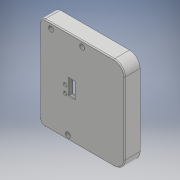
# Autodesk Inventor part: back
Saved by Autodesk Inventor 2017 (Build 210142000, 142)
## iProperties
Created: 2017-07-30
Part Number: back
Material: Generic
Document SubType Name: Modeling
Designer: Käyttäjä
Density: 1 g/cm^3
Appearance: Default
Author: Käyttäjä
Autodesk Inventor part; units mm, degrees
ref_plane "YZ Plane" through (0, 0, 0) normal (1, 0, 0) x (0, 1, 0)
ref_plane "XZ Plane" through (0, 0, 0) normal (0, 1, 0) x (-1, 0, 0)
ref_plane "XY Plane" through (0, 0, 0) normal (0, 0, 1) x (1, 0, 0)
sketch "Sketch1" plane through (0, 0, 0) normal (0, 1, 0) x (-1, 0, 0)
  line L0 (10, 0) -> (83, 0)
  line L1 (87, -4) -> (87, -92)
  line L2 (83, -96) -> (10, -96)
  line L3 (0, -86) -> (0, -10)
  arc A0 (10, 0) -> (0, -10) centre (10, -10) ccw
  arc A1 (0, -86) -> (10, -96) centre (10, -86) ccw
  arc A2 (87, -4) -> (83, 0) centre (83, -4) ccw
  arc A3 (83, -96) -> (87, -92) centre (83, -92) ccw
  line L4 (88.2, -92) -> (88.2, -4)
  arc A4 (88.2, -4) -> (83, 1.2) centre (83, -4) ccw
  line L5 (83, 1.2) -> (10, 1.2)
  arc A5 (10, 1.2) -> (-1.2, -10) centre (10, -10) ccw
  line L6 (-1.2, -10) -> (-1.2, -86)
  arc A6 (-1.2, -86) -> (10, -97.2) centre (10, -86) ccw
  line L7 (10, -97.2) -> (83, -97.2)
  arc A7 (83, -97.2) -> (88.2, -92) centre (83, -92) ccw
  point P0 (0, 0)
  point P1 (87, 0)
  point P2 (0, -96)
  dimension "d0" = 96
  dimension "d1" = 87
  dimension "d2" = 10
  dimension "d3" = 4
  dimension "d4" = 1.2
  constraints: 16 end point, 16 point on circle, 8 centre point, 8 tangent, 6 point on line, 4 parallel, 2 equal radius, 2 perpendicular, 1 horizontal, 7 other
  measures "d0" distance of point (0, -96) point (0, 0)
  measures "d1" distance of point (0, 0) point (87, 0)
  measures "d2" radius of A0
  measures "d3" radius of A2
  measures "d4" distance between parallel lines of L1 L4
extrude "walls" add sketch "Sketch1" along normal blind 15.5
sketch "Sketch2" plane through (0, 0, 0) normal (0, -1, 0) x (1, 0, 0)
  arc A0 (-83, 0) -> (-87, -4) centre (-83, -4) ccw projected
  line L0 (-83, 0) -> (-10, 0) projected
  arc A1 (0, -10) -> (-10, 0) centre (-10, -10) ccw projected
  line L1 (0, -10) -> (0, -86) projected
  arc A2 (-10, -96) -> (0, -86) centre (-10, -86) ccw projected
  line L2 (-10, -96) -> (-83, -96) projected
  arc A3 (-87, -92) -> (-83, -96) centre (-83, -92) ccw projected
  line L3 (-87, -92) -> (-87, -4) projected
  line L4 (-88.2, -92) -> (-88.2, -4) projected
  arc A4 (-88.2, -92) -> (-83, -97.2) centre (-83, -92) ccw projected
  line L5 (-10, -97.2) -> (-83, -97.2) projected
  arc A5 (-10, -97.2) -> (1.2, -86) centre (-10, -86) ccw projected
  line L6 (1.2, -10) -> (1.2, -86) projected
  arc A6 (1.2, -10) -> (-10, 1.2) centre (-10, -10) ccw projected
  line L7 (-83, 1.2) -> (-10, 1.2) projected
  arc A7 (-83, 1.2) -> (-88.2, -4) centre (-83, -4) ccw projected
  point P0 (0, 0)
extrude "back" add sketch "Sketch2" along normal blind 1 contours L0 A1 L1 A2 L2 A3 L3 A0 | L4 A7 L7 A6 L6 A5 L5 A4
sketch "Sketch3" plane through (-88.2, 15.5, -92) normal (-1, 0, 0) x (0, 0, 1)
  line L0 (0, -15.5) -> (88, -15.5) projected
  line L1 (92, -15.5) -> (92, 0) projected
  circle A0 centre (88, -5) radius 2
  line L2 (-4, -15.5) -> (-4, 0) projected
  circle A1 centre (0, -5) radius 2
  dimension "d9" = 4
  dimension "d10" = 4
  dimension "d11" = 10.5
  dimension "d12" = 4
  constraints: 2 centre point, 1 equal radius, 1 horizontal alignment
  measures "d9" distance from line of L1 A0.centre
  measures "d10" distance from line of A1.centre L2
  measures "d11" distance from line of L0 A0.centre
  measures "d12" diameter of A0
extrude "string holes" cut sketch "Sketch3" against normal up to next
sketch "Sketch5" plane through (0, 0, 0) normal (0, 1, 0) x (1, 0, 0)
  circle A0 centre (-76.5, 4.5) radius 2.75
  circle A1 centre (-58.5, 92.5) radius 2.75
  line L0 (0, 86) -> (0, 10) projected
  line L1 (-83, 96) -> (-10, 96) projected
  circle A2 centre (-43.5, 4.5) radius 2.75
  line L2 (-87, 4) -> (-87, 92) projected
  point P0 (0, 0)
  dimension "d19" = 5.5
  dimension "d22" = 3.5
  dimension "d23" = 91.5
  dimension "d130" = 10.5
  dimension "d131" = 33
  dimension "d132" = 15
  constraints: 3 centre point, 2 equal radius, 1 horizontal alignment
  measures "d19" diameter of A0
  measures "d22" distance from line of L1 A1.centre
  measures "d23" distance from line of A0.centre L1
  measures "d130" distance from line of L2 A0.centre
  measures "d131" distance of A2.centre A0.centre
  measures "d132" horizontal distance of A2.centre A1.centre
extrude "PCB pillars" add sketch "Sketch5" along normal blind 10.5
sketch "Sketch6" plane through (-10, 15.5, -97.2) normal (0, 0, -1) x (-1, 0, 0)
  line L0 (45, 0) -> (30, 0)
  line L1 (30, 0) -> (30, -8.5)
  line L2 (30, -8.5) -> (45, -8.5)
  line L3 (45, -8.5) -> (45, 0)
  line L4 (-10, -15.5) -> (-10, 0) projected
  line L5 (0, 0) -> (73, 0) projected
  line L6 (0, -15.5) -> (73, -15.5) projected
  line L7 (77, -15.5) -> (77, -7) projected
  dimension "d30" = 7
  dimension "d137" = 15
  dimension "d138" = 32
  constraints: 8 end point, 2 parallel, 1 horizontal, 1 perpendicular, 1 point on line
  measures "d30" distance between parallel lines of L2 L6
  measures "d137" distance of L1.end L2.end
  measures "d138" distance between parallel lines of L7 L3
sketch "Sketch7" plane through (-76.5, 10.5, -4.5) normal (0, 1, 0) x (1, 0, 0)
  circle A0 centre (0, 0) radius 2.75 projected
  circle A1 centre (0, 0) radius 1.75
  circle A2 centre (33, 0) radius 2.75 projected
  circle A3 centre (18, 88) radius 2.75 projected
  circle A4 centre (33, 0) radius 1.75
  circle A5 centre (18, 88) radius 1.75
  point P0 (76.5, -4.5)
  dimension "d31" = 3.5
  constraints: 3 centre point, 3 coincident, 2 equal radius
  measures "d31" diameter of A1
sketch "Sketch8" plane through (-88.2, 15.5, -92) normal (-1, 0, 0) x (0, 0, 1)
  line L0 (-4, -15.5) -> (-4, 0) projected
  line L1 (92, -15.5) -> (92, 0) projected
  line L2 (88, 0) -> (0, 0) projected
  line L3 (39, 0) -> (49, 0)
  line L4 (49, 0) -> (49, -10.1)
  line L5 (49, -10.1) -> (39, -10.1)
  line L6 (39, -10.1) -> (39, 0)
  line L7 (0, -15.5) -> (88, -15.5) projected
  point P0 (44, -15.5)
  point P1 (44, -10.1)
  dimension "d34" = 5.4
  dimension "d35" = 10
  constraints: 8 end point, 2 midpoint, 2 parallel, 1 horizontal, 1 perpendicular, 1 point on line, 1 vertical alignment
  measures "d34" distance between parallel lines of L7 L5
  measures "d35" distance of L4.end L5.end
extrude "Extrusion5" cut sketch "Sketch8" against normal blind 9.5
extrude "Extrusion6" cut sketch "Sketch7" against normal through all contours A1 | A4 | A5
sketch "Sketch9" plane through (0, 0, 0) normal (0, 1, 0) x (1, 0, 0)
  circle A0 centre (-76.5, 4.5) radius 1.75 projected
  circle A1 centre (-43.5, 4.5) radius 1.75 projected
  circle A2 centre (-58.5, 92.5) radius 1.75 projected
  circle A3 centre (-58.5, 92.5) radius 2.75 projected
  circle A4 centre (-76.5, 4.5) radius 2.75 projected
  circle A5 centre (-43.5, 4.5) radius 2.75 projected
  arc A6 (-87, 4) -> (-83, 0) centre (-83, 4) ccw projected
  line L0 (-83, 0) -> (-10, 0) projected
  arc A7 (-10, 0) -> (0, 10) centre (-10, 10) ccw projected
  line L1 (0, 10) -> (0, 86) projected
  arc A8 (0, 86) -> (-10, 96) centre (-10, 86) ccw projected
  line L2 (-10, 96) -> (-83, 96) projected
  arc A9 (-83, 96) -> (-87, 92) centre (-83, 92) ccw projected
  line L3 (-87, 92) -> (-87, 4) projected
  circle A10 centre (-43.5, 4.5) radius 2.75 projected
  circle A11 centre (-58.5, 92.5) radius 2.75 projected
  circle A12 centre (-76.5, 4.5) radius 5.7
  line L4 (-10, 0) -> (-83, 0) projected
  circle A13 centre (-43.5, 4.5) radius 5.7
  circle A14 centre (-58.5, 92.5) radius 4.7
  line L5 (-83, 96) -> (-10, 96) projected
  line L6 (-10, -1.2) -> (-83, -1.2) projected
  line L7 (-83, 97.2) -> (-10, 97.2) projected
  point P0 (0, 0)
  constraints: 3 centre point, 3 coincident, 2 tangent, 1 equal radius
extrude "Extrusion7" add sketch "Sketch9" along normal blind 3 contours A12 L0 | L0 A12 | A14 L2 | L2 A14 | A13 L0 | L0 A13
extrude "Extrusion8" cut sketch "Sketch6" against normal blind 3
fillet "Fillet3" radius 1 2 edges at (-87.6, 5.4, -53) (-87.6, 5.4, -43)
sketch "Sketch12" plane through (-58.5, 10.5, -92.5) normal (0, 1, 0) x (1, 0, 0)
  circle A0 centre (0, 0) radius 1.75 projected
  circle A1 centre (0, 0) radius 2.75 projected
  circle A2 centre (0, 0) radius 2.75 projected
  line L0 (-1.8, 2.0791) -> (-1.8, -2.0791)
  point P0 (58.5, -92.5)
  dimension "d57" = 1.8
  constraints: 4 point on circle, 2 end point, 1 vertical
  measures "d57" distance from line of L0 A0.centre
extrude "room for esp" cut sketch "Sketch12" against normal blind 2.5 contours L0 A1 picked at (-1.9501, -0.5269)
fillet "Fillet4" radius 2 3 edges at (-79.25, 3, -4.5) (-46.25, 3, -4.5) (-61.25, 3, -92.5)
sketch "Sketch13" plane through (0, -1, 0) normal (0, -1, 0) x (1, 0, 0)
  circle A0 centre (-43.5, -4.5) radius 1.75 projected
  circle A1 centre (-76.5, -4.5) radius 1.75 projected
  circle A2 centre (-58.5, -92.5) radius 1.75 projected
  line L0 (-88.2, -4) -> (-88.2, -92) projected
  arc A3 (-88.2, -92) -> (-83, -97.2) centre (-83, -92) ccw projected
  line L1 (-83, -97.2) -> (-10, -97.2) projected
  arc A4 (-10, -97.2) -> (1.2, -86) centre (-10, -86) ccw projected
  line L2 (1.2, -86) -> (1.2, -10) projected
  arc A5 (1.2, -10) -> (-10, 1.2) centre (-10, -10) ccw projected
  line L3 (-10, 1.2) -> (-83, 1.2) projected
  arc A6 (-83, 1.2) -> (-88.2, -4) centre (-83, -4) ccw projected
  circle A7 centre (-58.5, -92.5) radius 2.25
  circle A8 centre (-43.5, -4.5) radius 2.25
  circle A9 centre (-76.5, -4.5) radius 2.25
  point P0 (0, 0)
  dimension "d77" = 4.5
  dimension "d78" = 4.5
  dimension "d79" = 4.5
  constraints: 3 centre point, 3 coincident
  measures "d77" diameter of A7
  measures "d78" diameter of A9
  measures "d79" diameter of A8
extrude "inser holes" cut sketch "Sketch13" against normal blind 5 contours A7 | A8 | A9
fillet "Fillet6" radius 0.5 3 edges at (-60.75, -1, -92.5) (-78.75, -1, -4.5) (-45.75, -1, -4.5)
fillet "Fillet7" radius 1 8 edges at (-2.0804, -1, -93.9196) (1.2, -1, -48) (-2.0804, -1, -2.0804) (-46.5, -1, 1.2) (-86.677, -1, -0.323) (-88.2, -1, -48) (-86.677, -1, -95.677) (-46.5, -1, -97.2)
chamfer "Chamfer8" distance 0.5 angle 45 1 edges at (-60.75, 4, -92.5) measured on face at (-60.65, 4, -92.5)
chamfer "Chamfer9" distance 0.5 angle 45 1 edges at (-78.75, 4, -4.5) measured on face at (-78.65, 4, -4.5)
chamfer "Chamfer10" distance 0.5 angle 45 1 edges at (-45.75, 4, -4.5) measured on face at (-45.65, 4, -4.5)
fillet "Fillet11" radius 0.5 5 edges at (-88.2, 5.6929, -52.7071) (-88.2, 5.4, -48) (-88.2, 5.6929, -43.2929) (-88.2, 10.95, -43) (-88.2, 10.95, -53)
sketch "Sketch14" plane through (0, 0, 0) normal (0, 1, 0) x (1, 0, 0)
  arc A0 (-87.7, 43) -> (-88.2, 42.5) centre (-87.7, 42.5) ccw projected
  line L0 (-88.2, 42.5) -> (-88.2, 4) projected
  arc A1 (-88.2, 4) -> (-83, -1.2) centre (-83, 4) ccw projected
  line L1 (-83, -1.2) -> (-10, -1.2) projected
  arc A2 (-10, -1.2) -> (1.2, 10) centre (-10, 10) ccw projected
  line L2 (1.2, 10) -> (1.2, 86) projected
  arc A3 (1.2, 86) -> (-10, 97.2) centre (-10, 86) ccw projected
  line L3 (-10, 97.2) -> (-40, 97.2) projected
  line L4 (-40, 97.2) -> (-40, 96) projected
  line L5 (-40, 96) -> (-10, 96) projected
  arc A4 (0, 86) -> (-10, 96) centre (-10, 86) ccw projected
  line L6 (0, 86) -> (0, 10) projected
  arc A5 (-10, 0) -> (0, 10) centre (-10, 10) ccw projected
  line L7 (-10, 0) -> (-83, 0) projected
  arc A6 (-87, 4) -> (-83, 0) centre (-83, 4) ccw projected
  line L8 (-87, 4) -> (-87, 43) projected
  line L9 (-87, 43) -> (-87.7, 43) projected
  line L10 (-57.5, 40) -> (-51.5, 40)
  line L11 (-51.5, 40) -> (-51.5, 56)
  line L12 (-51.5, 56) -> (-57.5, 56)
  line L13 (-57.5, 56) -> (-57.5, 40)
  line L14 (0, 86) -> (0, 10) projected
  point P0 (0, 0)
  point P1 (-57.5, 48)
  point P2 (0, 48)
  dimension "d105" = 16
  dimension "d133" = 29.5
  dimension "d134" = 6
  constraints: 8 end point, 2 midpoint, 2 parallel, 1 horizontal, 1 horizontal alignment, 1 perpendicular
  measures "d105" distance of L12.end L10.start
  measures "d133" distance between parallel lines of L8 L13
  measures "d134" distance of L10.start L10.end
extrude "connector hole" cut sketch "Sketch14" against normal blind 5 contours L13 L12 L11 L10
fillet "Fillet13" radius 0.5 6 edges at (-87.8, 10.5005, -94) (-88.2, 9.0858, -90.5858) (-88.2, 11.9142, -90.5858) (-88.2, 10.5, -6) (-87.9774, 9.1829, -2.4949) (-87.9773, 11.8167, -2.4946)
sketch "Sketch16" plane through (0, 0, 0) normal (0, 1, 0) x (1, 0, 0)
  line L0 (-51.5, 56) -> (-51.5, 40) projected
  line L1 (-51.5, 40) -> (-57.5, 40) projected
  line L2 (-57.5, 40) -> (-57.5, 56) projected
  line L3 (-57.5, 56) -> (-51.5, 56) projected
  arc A0 (-40.0014, 0) -> (-46.9986, 0) centre (-43.5, 4.5) ccw projected
  line L4 (-40.0014, 0) -> (-10, 0) projected
  arc A1 (-10, 0) -> (0, 10) centre (-10, 10) ccw projected
  line L5 (0, 10) -> (0, 86) projected
  arc A2 (0, 86) -> (-10, 96) centre (-10, 86) ccw projected
  line L6 (-10, 96) -> (-55.3631, 96) projected
  arc A3 (-61.6369, 96) -> (-55.3631, 96) centre (-58.5, 92.5) ccw projected
  line L7 (-61.6369, 96) -> (-83, 96) projected
  arc A4 (-83, 96) -> (-87, 92) centre (-83, 92) ccw projected
  line L8 (-87, 92) -> (-87, 4) projected
  arc A5 (-87, 4) -> (-83, 0) centre (-83, 4) ccw projected
  line L9 (-83, 0) -> (-79.9986, 0) projected
  arc A6 (-73.0014, 0) -> (-79.9986, 0) centre (-76.5, 4.5) ccw projected
  line L10 (-73.0014, 0) -> (-46.9986, 0) projected
  line L11 (-59.5, 58) -> (-59.5, 38)
  line L12 (-59.5, 38) -> (-49.5, 38)
  line L13 (-49.5, 38) -> (-49.5, 58)
  line L14 (-49.5, 58) -> (-59.5, 58)
  point P0 (0, 0)
  dimension "d110" = 2
  constraints: 8 end point, 3 other
  measures "d110" distance between parallel lines of L2 L11
extrude "connector" add sketch "Sketch16" along normal blind 3 contours L14 L13 L12 L11
sketch "Sketch17" plane through (0, 0, 0) normal (0, 1, 0) x (1, 0, 0)
  circle A0 centre (-61.5, 48) radius 1.5
  circle A1 centre (-61.5, 56) radius 1.5
  line L0 (0, 86) -> (0, 10) projected
  line L1 (-83, 96) -> (-55, 96) projected
  line L2 (-87, 53) -> (-87, 92) projected
  point P0 (0, 0)
  dimension "d113" = 3
  dimension "d115" = 40
  dimension "d116" = 48
  dimension "d135" = 25.5
  constraints: 2 centre point, 1 equal radius, 1 vertical alignment
  measures "d113" diameter of A1
  measures "d115" distance from line of A1.centre L1
  measures "d116" distance from line of L1 A0.centre
  measures "d135" distance from line of A1.centre L2
extrude "buttons hole" cut sketch "Sketch17" against normal through all
sketch "Sketch18" plane through (0, 0, 0) normal (0, 1, 0) x (1, 0, 0)
  circle A0 centre (-61.5, 48) radius 1.5 projected
  circle A1 centre (-61.5, 56) radius 1.5 projected
  circle A2 centre (-61.5, 48) radius 2.5
  circle A3 centre (-61.5, 56) radius 2.5
  point P0 (0, 0)
  dimension "d119" = 5
  dimension "d120" = 5
  constraints: 2 centre point, 2 coincident
  measures "d119" diameter of A2
  measures "d120" diameter of A3
extrude "Extrusion18" add sketch "Sketch18" along normal blind 3
sketch "Sketch19" plane through (0, 0, 0) normal (0, 1, 0) x (1, 0, 0)
  arc A0 (-40.0014, 0) -> (-46.9986, 0) centre (-43.5, 4.5) ccw projected
  line L0 (-40.0014, 0) -> (-10, 0) projected
  arc A1 (-10, 0) -> (0, 10) centre (-10, 10) ccw projected
  line L1 (0, 10) -> (0, 86) projected
  arc A2 (0, 86) -> (-10, 96) centre (-10, 86) ccw projected
  line L2 (-10, 96) -> (-55.3631, 96) projected
  arc A3 (-61.6369, 96) -> (-55.3631, 96) centre (-58.5, 92.5) ccw projected
  line L3 (-61.6369, 96) -> (-83, 96) projected
  arc A4 (-83, 96) -> (-87, 92) centre (-83, 92) ccw projected
  line L4 (-87, 92) -> (-87, 4) projected
  arc A5 (-87, 4) -> (-83, 0) centre (-83, 4) ccw projected
  line L5 (-83, 0) -> (-79.9986, 0) projected
  arc A6 (-73.0014, 0) -> (-79.9986, 0) centre (-76.5, 4.5) ccw projected
  line L6 (-73.0014, 0) -> (-46.9986, 0) projected
  arc A7 (-59.5, 49.5) -> (-59.5, 46.5) centre (-61.5, 48) ccw projected
  line L7 (-59.5, 49.5) -> (-59.5, 54.5) projected
  arc A8 (-59.5, 57.5) -> (-59.5, 54.5) centre (-61.5, 56) ccw projected
  line L8 (-59.5, 57.5) -> (-59.5, 58) projected
  line L9 (-59.5, 58) -> (-49.5, 58) projected
  line L10 (-49.5, 58) -> (-49.5, 38) projected
  line L11 (-49.5, 38) -> (-59.5, 38) projected
  line L12 (-59.5, 38) -> (-59.5, 46.5) projected
  arc A9 (-10, 1.5) -> (-1.5, 10) centre (-10, 10) ccw
  arc A10 (-1.5, 86) -> (-10, 94.5) centre (-10, 86) ccw
  line L13 (-10, 1.5) -> (-10, 0)
  line L14 (-1.5, 10) -> (0, 10)
  line L15 (-10, 94.5) -> (-10, 96)
  line L16 (-1.5, 86) -> (0, 86)
  line L17 (0, 86) -> (0, 10) projected
  line L18 (0, 43) -> (-1.5, 43)
  line L19 (-1.5, 43) -> (-1.5, 53)
  line L20 (-1.5, 53) -> (0, 53)
  line L21 (0, 53) -> (0, 43)
  line L22 (1.2, 10) -> (1.2, 86) projected
  point P0 (0, 0)
  point P1 (1.2, 48)
  point P2 (-1.5, 48)
  dimension "d123" = 1.5
  dimension "d124" = 1.5
  dimension "d125" = 1.5
  dimension "d126" = 10
  constraints: 16 end point, 4 point on circle, 3 perpendicular, 2 centre point, 2 coincident, 2 horizontal, 2 midpoint, 2 parallel, 1 horizontal alignment, 1 point on line, 1 vertical
  measures "d123" radial gap between concentric circles of A10 A2
  measures "d124" radial gap between concentric circles of A9 A1
  measures "d125" distance of L18.start L18.end
  measures "d126" distance of L18.end L19.end
extrude "Extrusion19" add sketch "Sketch19" along normal up to surface (10.5 mm away) contours L13 A9 L14 A1 | L18 L19 L20 L1 | L16 A10 L15 A2
fillet "Fillet14" radius 2 9 edges at (-32.6816, 0, -96) (0, 0, -69.5) (-25.0007, 0, 0) (-60, 0, 0) (-81.4993, 0, 0) (-87, 0, -48) (-85.8284, 0, -94.8284) (-72.3184, 0, -96) (-85.8284, 0, -1.1716)
fillet "Fillet15" radius 0.5 6 edges at (-51.5, -1, -48) (-54.5, -1, -56) (-57.5, -1, -48) (-54.5, -1, -40) (-63, -1, -48) (-63, -1, -56)
body "Solid1"
